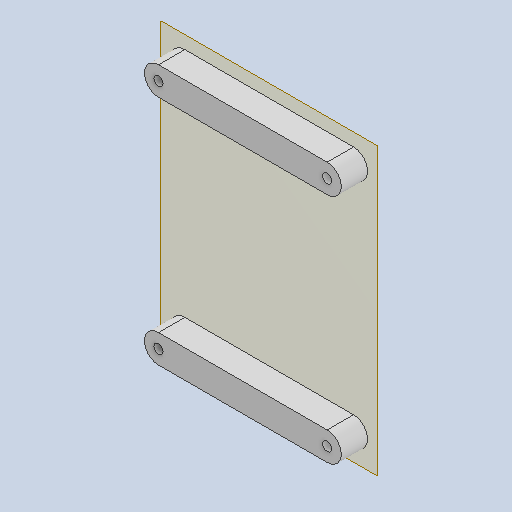
# Autodesk Inventor part: Oled Mount
Saved by Autodesk Inventor 2023 (Build 270158000, 158)
## iProperties
Created: 2023-06-04
Part Number: Oled Mount
Material: Generic
Document SubType Name: Modeling
Designer: jeffb
Density: 1 g/cm^3
Appearance: Default
Author: jeffb
Autodesk Inventor part; units mm, degrees
ref_plane "YZ Plane" through (0, 0, 0) normal (1, 0, 0) x (0, 1, 0)
ref_plane "XZ Plane" through (0, 0, 0) normal (0, 1, 0) x (-1, 0, 0)
ref_plane "XY Plane" through (0, 0, 0) normal (0, 0, 1) x (1, 0, 0)
ref_plane "Work Plane1" through (0, 0, 0) normal (0, 0, 1) x (1, 0, 0)
sketch "Sketch1" plane through (0, 0, 0) normal (0, 0, 1) x (1, 0, 0)
  circle A0 centre (-15.24, -20.955) radius 1.25 construction
  circle A1 centre (15.24, -20.955) radius 1.25 construction
  circle A2 centre (15.24, 20.955) radius 1.25 construction
  circle A3 centre (-15.24, 20.955) radius 1.25 construction
  circle A4 centre (-15.24, 20.955) radius 0.8255
  circle A5 centre (15.24, 20.955) radius 0.8255
  circle A6 centre (-15.24, -20.955) radius 0.8255
  circle A7 centre (15.24, -20.955) radius 0.8255
  line L0 (-15.24, 20.955) -> (15.24, 20.955) construction
  line L1 (-15.24, 18.415) -> (15.24, 18.415)
  line L2 (15.24, 23.495) -> (-15.24, 23.495)
  arc A8 (-15.24, 23.495) -> (-15.24, 18.415) centre (-15.24, 20.955) ccw
  arc A9 (15.24, 18.415) -> (15.24, 23.495) centre (15.24, 20.955) ccw
  line L3 (-15.24, -20.955) -> (15.24, -20.955) construction
  line L4 (-15.24, -23.495) -> (15.24, -23.495)
  line L5 (15.24, -18.415) -> (-15.24, -18.415)
  arc A10 (-15.24, -18.415) -> (-15.24, -23.495) centre (-15.24, -20.955) ccw
  arc A11 (15.24, -23.495) -> (15.24, -18.415) centre (15.24, -20.955) ccw
  point P0 (0, 0)
  point P1 (0, 20.955)
  point P2 (0, -20.955)
  dimension "d0" = 1.651
  dimension "d1" = 5.08
  dimension "d2" = 5.08
  constraints: 16 end point, 8 centre point, 8 point on circle, 8 tangent, 4 coincident, 3 equal radius, 3 parallel, 2 midpoint, 1 horizontal
  measures "d0" diameter of A4
  measures "d1" diameter of A9
  measures "d2" diameter of A11
extrude "Extrusion1" add sketch "Sketch1" along normal blind 4.7625
body "Solid1"
